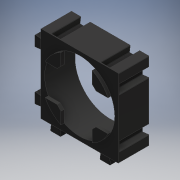
# Autodesk Inventor part: Base_18650
Saved by Autodesk Inventor 2018.3 (Build 223285000, 285)
## iProperties
Created: 2020-11-27
Part Number: Base_18650
Material: Goma
Document SubType Name: Modeling
Designer: felip
Density: 0.93 g/cm^3
Appearance: Goma - Negro
Author: felip
Autodesk Inventor part; units mm, degrees
ref_plane "YZ Plane" through (0, 0, 0) normal (1, 0, 0) x (0, 1, 0)
ref_plane "XZ Plane" through (0, 0, 0) normal (0, 1, 0) x (-1, 0, 0)
ref_plane "XY Plane" through (0, 0, 0) normal (0, 0, 1) x (1, 0, 0)
sketch "Boceto1" plane through (0, 0, 0) normal (0, 1, 0) x (-1, 0, 0)
  circle A0 centre (0, 0) radius 9
  line L0 (0, 0) -> (10, -10) construction
  line L1 (10, 10) -> (-10, -10) construction
  line L2 (-10, 9.9) -> (-10, 7.6125)
  line L3 (-8.3, 6.35) -> (-8.3, 5.1125)
  line L4 (-8.4117, 7.6869) -> (-9.8883, 7.5131)
  line L5 (-8.4117, 5.0131) -> (-9.8883, 5.1869)
  line L6 (-8.3, -6.35) -> (-8.3, -5.1125)
  line L7 (-8.4117, -7.6869) -> (-9.8883, -7.5131)
  line L8 (-8.4117, -5.0131) -> (-9.8883, -5.1869)
  line L9 (-7.6869, 8.4117) -> (-7.5131, 9.8883)
  line L10 (-5.0131, 8.4117) -> (-5.1869, 9.8883)
  line L11 (5.0131, 8.4117) -> (5.1869, 9.8883)
  line L12 (6.35, 8.3) -> (5.1125, 8.3)
  line L13 (7.6869, 8.4117) -> (7.5131, 9.8883)
  line L14 (-5.0131, -11.5883) -> (-5.1869, -10.1117)
  line L15 (-7.6869, -11.5883) -> (-7.5131, -10.1117)
  line L16 (-5.1125, -11.7) -> (-7.5875, -11.7)
  line L17 (7.6869, -11.5883) -> (7.5131, -10.1117)
  line L18 (5.1125, -11.7) -> (7.5875, -11.7)
  line L19 (5.0131, -11.5883) -> (5.1869, -10.1117)
  line L20 (11.5883, -5.0131) -> (10.1117, -5.1869)
  line L21 (11.7, -5.1125) -> (11.7, -7.5875)
  line L22 (11.5883, -7.6869) -> (10.1117, -7.5131)
  line L23 (11.5883, 7.6869) -> (10.1117, 7.5131)
  line L24 (11.5883, 5.0131) -> (10.1117, 5.1869)
  line L25 (11.7, 5.1125) -> (11.7, 7.5875)
  line L26 (10, 9.9) -> (10, 7.6125)
  arc A1 (11.7, 7.5875) -> (11.5883, 7.6869) centre (11.6, 7.5875) ccw
  arc A2 (11.5883, 5.0131) -> (11.7, 5.1125) centre (11.6, 5.1125) ccw
  arc A3 (10, 7.6125) -> (10.1117, 7.5131) centre (10.1, 7.6125) ccw
  arc A4 (10.1117, 5.1869) -> (10, 5.0875) centre (10.1, 5.0875) ccw
  line L27 (10, 5.0875) -> (10, -5.0875)
  line L28 (10, -7.6125) -> (10, -9.9)
  arc A5 (10, -5.0875) -> (10.1117, -5.1869) centre (10.1, -5.0875) ccw
  arc A6 (11.7, -5.1125) -> (11.5883, -5.0131) centre (11.6, -5.1125) ccw
  arc A7 (11.5883, -7.6869) -> (11.7, -7.5875) centre (11.6, -7.5875) ccw
  arc A8 (10.1117, -7.5131) -> (10, -7.6125) centre (10.1, -7.6125) ccw
  line L29 (9.9, -10) -> (7.6125, -10)
  line L30 (5.0875, -10) -> (-5.0875, -10)
  line L31 (-7.6125, -10) -> (-9.9, -10)
  arc A9 (5.1869, -10.1117) -> (5.0875, -10) centre (5.0875, -10.1) ccw
  arc A10 (5.0131, -11.5883) -> (5.1125, -11.7) centre (5.1125, -11.6) ccw
  arc A11 (7.5875, -11.7) -> (7.6869, -11.5883) centre (7.5875, -11.6) ccw
  arc A12 (7.6125, -10) -> (7.5131, -10.1117) centre (7.6125, -10.1) ccw
  arc A13 (-5.0875, -10) -> (-5.1869, -10.1117) centre (-5.0875, -10.1) ccw
  arc A14 (-5.1125, -11.7) -> (-5.0131, -11.5883) centre (-5.1125, -11.6) ccw
  arc A15 (-7.6869, -11.5883) -> (-7.5875, -11.7) centre (-7.5875, -11.6) ccw
  arc A16 (-7.5131, -10.1117) -> (-7.6125, -10) centre (-7.6125, -10.1) ccw
  line L32 (-10, -9.9) -> (-10, -7.6125)
  arc A17 (-10, -5.0875) -> (-9.8883, -5.1869) centre (-9.9, -5.0875) ccw
  arc A18 (-8.3, -5.1125) -> (-8.4117, -5.0131) centre (-8.4, -5.1125) ccw
  arc A19 (-8.4117, -7.6869) -> (-8.3, -7.5875) centre (-8.4, -7.5875) ccw
  arc A20 (-9.8883, -7.5131) -> (-10, -7.6125) centre (-9.9, -7.6125) ccw
  line L33 (-8.3, -6.35) -> (-8.3, -7.5875)
  line L34 (7.6125, 10) -> (9.9, 10)
  arc A21 (7.6125, 10) -> (7.5131, 9.8883) centre (7.6125, 9.9) ccw
  arc A22 (7.5875, 8.3) -> (7.6869, 8.4117) centre (7.5875, 8.4) ccw
  arc A23 (5.0131, 8.4117) -> (5.1125, 8.3) centre (5.1125, 8.4) ccw
  line L35 (6.35, 8.3) -> (7.5875, 8.3)
  line L36 (-9.9, 10) -> (-7.6125, 10)
  line L37 (-5.0875, 10) -> (5.0875, 10)
  line L38 (-7.5875, 8.3) -> (-5.1125, 8.3)
  arc A24 (-5.0875, 10) -> (-5.1869, 9.8883) centre (-5.0875, 9.9) ccw
  arc A25 (-5.1125, 8.3) -> (-5.0131, 8.4117) centre (-5.1125, 8.4) ccw
  arc A26 (-7.5131, 9.8883) -> (-7.6125, 10) centre (-7.6125, 9.9) ccw
  arc A27 (-7.6869, 8.4117) -> (-7.5875, 8.3) centre (-7.5875, 8.4) ccw
  line L39 (-10, -5.0875) -> (-10, 5.0875)
  line L40 (-10, 7.5) -> (-10, 10)
  line L41 (-8.3, 7.3529) -> (-8.3, 7.5875)
  line L42 (-8.3, 7.3529) -> (-8.3, 6.35)
  arc A28 (-8.3, 7.5875) -> (-8.4117, 7.6869) centre (-8.4, 7.5875) ccw
  arc A29 (-10, 7.6125) -> (-9.8883, 7.5131) centre (-9.9, 7.6125) ccw
  arc A30 (-9.8883, 5.1869) -> (-10, 5.0875) centre (-9.9, 5.0875) ccw
  arc A31 (-8.4117, 5.0131) -> (-8.3, 5.1125) centre (-8.4, 5.1125) ccw
  arc A32 (10, 9.9) -> (9.9, 10) centre (9.9, 9.9) ccw
  arc A33 (9.9, -10) -> (10, -9.9) centre (9.9, -9.9) ccw
  arc A34 (-10, -9.9) -> (-9.9, -10) centre (-9.9, -9.9) ccw
  arc A35 (-9.9, 10) -> (-10, 9.9) centre (-9.9, 9.9) ccw
  arc A36 (5.1869, 9.8883) -> (5.0875, 10) centre (5.0875, 9.9) ccw
  point P0 (0, 0)
  point P1 (-10, 5.2)
  point P2 (-8.3, 7.7)
  point P3 (-10, -5.2)
  point P4 (-10, -7.5)
  point P5 (-8.3, -7.7)
  point P6 (5.2, 10)
  point P7 (7.7, 8.3)
  point P8 (-7.5, -10)
  point P9 (7.5, -10)
  point P10 (5.2, -10)
  point P11 (7.7, -11.7)
  point P12 (5, -11.7)
  point P13 (11.7, -5)
  point P14 (10, -5.2)
  point P15 (11.7, -7.7)
  point P16 (10, -7.5)
  point P17 (-5.2, -10)
  dimension "d0" = 18
  dimension "d1" = 20
  dimension "d2" = 20
  dimension "d3" = 2.5
  dimension "d4" = 2.3
  dimension "d8" = 0.1
  dimension "d9" = 0.1
  dimension "d10" = 0.1
  dimension "d11" = 0.1
  dimension "d12" = 0.1
  dimension "d13" = 0.1
  dimension "d14" = 0.1
  dimension "d15" = 0.1
  dimension "d16" = 0.1
  dimension "d17" = 0.1
  dimension "d18" = 0.1
  dimension "d19" = 0.1
  dimension "d43" = 0.1
  constraints: 87 end point, 72 point on circle, 72 tangent, 45 point on line, 37 centre point, 23 equal radius, 18 parallel, 9 perpendicular, 6 symmetric about line, 5 horizontal, 3 vertical, 1 coincident, 1 midpoint
  measures "d0" diameter of A0
  measures "d1" distance of L0.end L1.end
  measures "d2" distance of L1.start L0.end
  measures "d3" distance of L40.end L40.start
  measures "d4" distance of L40.start point (-10, 5.2)
  measures "d8" radius of A1
  measures "d9" radius of A2
  measures "d10" radius of A3
  measures "d11" radius of A4
  measures "d12" radius of A5
  measures "d13" radius of A9
  measures "d14" radius of A17
  measures "d15" radius of A21
  measures "d16" radius of A24
  measures "d17" radius of A28
  measures "d18" radius of A32
  measures "d19" radius of A35
  measures "d43" radius of A36
extrude "Extrusión1" add sketch "Boceto1" along normal blind 7.8
sketch "Boceto2" plane through (0, 0, 0) normal (0, -1, 0) x (1, 0, 0)
  line L0 (5.1125, 8.3) -> (7.5875, 8.3) projected
  line L1 (6.35, 8.3) -> (7.7, 8.3)
  line L2 (6.35, 8.3) -> (5, 8.3)
  line L3 (6.35, 8.3) -> (6.35, 10)
  line L4 (6.35, 10) -> (7.7, 10)
  line L5 (7.6125, 10) -> (9.9, 10) projected
  line L6 (7.7, 8.3) -> (7.7, 10)
  line L7 (5, 8.3) -> (5, 10)
  line L8 (5, 10) -> (6.35, 10)
  point P0 (0, 0)
  dimension "d22" = 1.35
  dimension "d23" = 1.35
  dimension "d24" = 1.7
  constraints: 14 end point, 3 point on line, 2 perpendicular, 1 collinear, 1 midpoint, 1 parallel, 1 vertical
  measures "d22" distance of L1.start L1.end
  measures "d23" distance of L1.start L2.end
  measures "d24" distance of L1.start L3.end
extrude "Extrusión2" add sketch "Boceto2" against normal blind 0.2
sketch "Boceto3" plane through (0, 0, 0) normal (0, -1, 0) x (1, 0, 0)
  line L0 (-9.9, 10) -> (-7.6125, 10) projected
  line L1 (-8.0303, 10) -> (-4.8001, 10)
  line L2 (-4.8001, 10) -> (-4.8001, 8.1465)
  line L3 (-4.8001, 8.1465) -> (-8.0303, 8.1465)
  line L4 (-8.0303, 8.1465) -> (-8.0303, 10)
  line L5 (10, 9.9) -> (10, 7.6125) projected
  line L6 (10, 8.1465) -> (8.0988, 8.1465)
  line L7 (8.0988, 8.1465) -> (8.0988, 4.6857)
  line L8 (8.0988, 4.6857) -> (10, 4.6857)
  line L9 (10, 4.6857) -> (10, 8.1465)
  line L10 (10, 5.0875) -> (10, -5.0875) projected
  line L11 (10, -4.5899) -> (8.0988, -4.5899)
  line L12 (8.0988, -4.5899) -> (8.0988, -8.0513)
  line L13 (8.0988, -8.0513) -> (10, -8.0513)
  line L14 (10, -8.0513) -> (10, -4.5899)
  point P0 (0, 0)
  constraints: 24 end point, 6 parallel, 4 point on line, 3 horizontal, 3 perpendicular
extrude "Extrusión3" add sketch "Boceto3" against normal blind 0.2
sketch "Boceto4" plane through (0, 0, 0) normal (0, -1, 0) x (1, 0, 0)
  line L0 (9.9, -10) -> (7.6125, -10) projected
  line L1 (8.0587, -10) -> (4.5937, -10)
  line L2 (4.5937, -10) -> (4.5937, -11.8621)
  line L3 (4.5937, -11.8621) -> (8.0587, -11.8621)
  line L4 (8.0587, -11.8621) -> (8.0587, -10)
  line L5 (5.0875, -10) -> (-5.0875, -10) projected
  line L6 (-4.2911, -10) -> (-8.2093, -10)
  line L7 (-8.2093, -10) -> (-8.2093, -11.8621)
  line L8 (-8.2093, -11.8621) -> (-4.2911, -11.8621)
  line L9 (-4.2911, -11.8621) -> (-4.2911, -10)
  line L10 (-10, -9.9) -> (-10, -7.6125) projected
  line L11 (-10, -8.4914) -> (-12.1328, -8.4914)
  line L12 (-12.1328, -8.4914) -> (-12.1328, -3.8938)
  line L13 (-12.1328, -3.8938) -> (-10, -3.8938)
  line L14 (-10, -3.8938) -> (-10, -8.4914)
  line L15 (-10, 7.6125) -> (-10, 9.9) projected
  line L16 (-10, 8.328) -> (-12.1328, 8.328)
  line L17 (-12.1328, 8.328) -> (-12.1328, 4.1194)
  line L18 (-12.1328, 4.1194) -> (-10, 4.1194)
  line L19 (-10, 4.1194) -> (-10, 8.328)
  point P0 (0, 0)
  constraints: 32 end point, 8 parallel, 6 point on line, 4 horizontal, 4 perpendicular
extrude "Extrusión4" cut sketch "Boceto4" against normal blind 0.2
sketch "Boceto5" plane through (0, 0, 0) normal (0, -1, 0) x (1, 0, 0)
  circle A0 centre (0, 0) radius 9 projected
  line L0 (-4, -8.0623) -> (-4, -5)
  line L1 (-5, -4) -> (-8.0623, -4)
  line L2 (-4, 8.0623) -> (-4, 5)
  line L3 (-5, 4) -> (-8.0623, 4)
  line L4 (4, -8.0623) -> (4, -5)
  line L5 (5, -4) -> (8.0623, -4)
  line L6 (4, 8.0623) -> (4, 5)
  line L7 (5, 4) -> (8.0623, 4)
  line L8 (-4, -5) -> (-5, -4)
  line L9 (-5, 4) -> (-4, 5)
  line L10 (4, 5) -> (5, 4)
  line L11 (5, -4) -> (4, -5)
  arc A1 (4, -8.0623) -> (8.0623, -4) centre (0, 0) ccw
  arc A2 (8.0623, 4) -> (4, 8.0623) centre (0, 0) ccw
  arc A3 (-4, 8.0623) -> (-8.0623, 4) centre (0, 0) ccw
  arc A4 (-8.0623, -4) -> (-4, -8.0623) centre (0, 0) ccw
  point P0 (0, -9)
  point P1 (-4, -4)
  point P2 (-4, -10)
  point P3 (-10, -4)
  point P4 (-9, 0)
  point P5 (-4, 4)
  point P6 (-4, 10)
  point P7 (-10, 4)
  point P8 (4, -4)
  point P9 (4, -10)
  point P10 (10, -4)
  point P11 (4, 10)
  point P12 (4, 4)
  point P13 (10, 4)
  dimension "d31" = 6
  dimension "d32" = 6
  dimension "d33" = 1
  dimension "d34" = 1
  dimension "d35" = 1
  dimension "d36" = 1
  dimension "d37" = 1
  dimension "d38" = 1
  dimension "d39" = 1
  dimension "d40" = 1
  constraints: 24 end point, 14 point on circle, 8 point on line, 4 centre point, 1 coincident
  measures "d31" distance of point (-10, -4) point (-4, -4)
  measures "d32" distance of point (-4, -10) point (-4, -4)
  measures "d33" distance of L0.end point (-4, -4)
  measures "d34" distance of L1.start point (-4, -4)
  measures "d35" distance of L3.start point (-4, 4)
  measures "d36" distance of L2.end point (-4, 4)
  measures "d37" distance of L6.end point (4, 4)
  measures "d38" distance of L7.start point (4, 4)
  measures "d39" distance of L5.start point (4, -4)
  measures "d40" distance of L4.end point (4, -4)
extrude "Extrusión5" add sketch "Boceto5" along normal blind 0.8 contours L7 L10 L6 A0 | A0 L4 L11 L5 | L2 L9 L3 A0 | A0 L1 L8 L0
equation "\"d34\" = d33"
equation "\"d35\" = d33"
equation "\"d36\" = d35"
equation "\"d37\" = d33"
equation "\"d38\" = d37"
equation "\"d39\" = d33"
equation "\"d40\" = d39"
